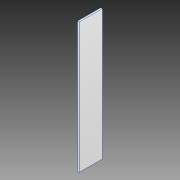
# Autodesk Inventor part: FE-130-001 End Platet
Saved by Autodesk Inventor 2021 (Build 250183000, 183)
## iProperties
Created: 2021-01-11
Part Number: FE-130-001 End Platet
Material: Aluminum 6061
Document SubType Name: Modeling
Density: 2.7 g/cm^3
Appearance: Aluminum - Flat
Autodesk Inventor part; units mm, degrees
ref_plane "YZ Plane" through (0, 0, 0) normal (1, 0, 0) x (0, 1, 0)
ref_plane "XZ Plane" through (0, 0, 0) normal (0, 1, 0) x (-1, 0, 0)
ref_plane "XY Plane" through (0, 0, 0) normal (0, 0, 1) x (1, 0, 0)
sketch "Sketch1" plane through (0, 0, 0) normal (1, 0, 0) x (0, 1, 0)
  line L0 (-250.825, 44.45) -> (250.825, 44.45)
  line L1 (250.825, 44.45) -> (250.825, -44.45)
  line L2 (250.825, -44.45) -> (-250.825, -44.45)
  line L3 (-250.825, -44.45) -> (-250.825, 44.45)
  line L4 (-250.825, 44.45) -> (250.825, -44.45) construction
  line L5 (250.825, 44.45) -> (-250.825, -44.45) construction
  point P0 (0, 0)
  dimension "d0" = 501.65
  dimension "d1" = 88.9
  constraints: 12 end point, 2 midpoint, 2 parallel, 1 horizontal, 1 perpendicular
  measures "d0" distance of L1.end L2.end
  measures "d1" distance of L0.end L1.end
extrude "Extrusion1" add sketch "Sketch1" along normal blind 6.35
body "Solid1"
